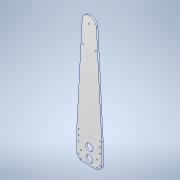
# Autodesk Inventor part: 関節3_側板1
Saved by Autodesk Inventor 2021 (Build 250183000, 183)
## iProperties
Created: 2022-01-31
Part Number: 関節3_側板1
Material: アルミニウム 6061
Document SubType Name: Modeling
Designer: hirohumi
Density: 2.7 g/cm^3
Appearance: アルミニウム - フラット
Author: hirohumi
Autodesk Inventor part; units mm, degrees
ref_plane "YZ Plane" through (0, 0, 0) normal (1, 0, 0) x (0, 1, 0)
ref_plane "XZ Plane" through (0, 0, 0) normal (0, 1, 0) x (-1, 0, 0)
ref_plane "XY Plane" through (0, 0, 0) normal (0, 0, 1) x (1, 0, 0)
sketch "スケッチ1" plane through (0, 0, 0) normal (0, 0, 1) x (1, 0, 0)
  circle A0 centre (0, 0) radius 10
  circle A1 centre (0, 0) radius 50 construction
  circle A2 centre (0, -28) radius 11.9375 construction
  circle A3 centre (-0.2119, 34.8748) radius 11.9375 construction
  circle A4 centre (0, -28) radius 15.9375 construction
  circle A5 centre (0, 0) radius 4 construction
  circle A6 centre (0, -28) radius 22.5 construction
  circle A7 centre (0, 300) radius 5 construction
  circle A8 centre (0, 300) radius 47.7465 construction
  line L0 (47.4611, 294.7873) -> (11.8661, -29.3033) construction
  line L1 (-47.4611, 294.7873) -> (-11.8661, -29.3033) construction
  circle A9 centre (-0.2119, 34.8748) radius 19.25 construction
  line L2 (-12.0776, 316.763) -> (11.6547, 316.763) construction
  line L3 (-22.6185, -92.0395) -> (22.1946, -92.0395) construction
  line L4 (22.5, -18) -> (-22.5, -18) construction
  line L5 (-22.5, -18) -> (-22.5, -38) construction
  line L6 (-22.5, -38) -> (22.5, -38) construction
  line L7 (22.5, -38) -> (22.5, -18) construction
  line L8 (22.5, -18) -> (-22.5, -38) construction
  line L9 (-22.5, -18) -> (22.5, -38) construction
  circle A10 centre (-22.5, -18) radius 1.6
  circle A11 centre (22.5, -18) radius 1.6
  circle A12 centre (22.5, -38) radius 1.6
  circle A13 centre (-22.5, -38) radius 1.6
  line L10 (30, 30) -> (-30, 30) construction
  line L11 (-30, 30) -> (-30, -30) construction
  line L12 (-30, -30) -> (30, -30) construction
  line L13 (30, -30) -> (30, 30) construction
  line L14 (30, 30) -> (-30, -30) construction
  line L15 (-30, 30) -> (30, -30) construction
  circle A14 centre (-30, 30) radius 1.25
  circle A15 centre (30, 30) radius 1.25
  circle A16 centre (30, -30) radius 1.25
  circle A17 centre (-30, -30) radius 1.25
  circle A18 centre (0, -28) radius 10
  circle A19 centre (0, 300) radius 1.75
  arc A20 (35, 30) -> (34.9923, 30.2769) centre (30, 30) ccw
  arc A21 (33.6477, -33.4197) -> (35, -30) centre (30, -30) ccw
  arc A22 (22.5, -43) -> (26.1477, -41.4197) centre (22.5, -38) ccw
  arc A23 (-26.1477, -41.4197) -> (-22.5, -43) centre (-22.5, -38) ccw
  arc A24 (-35, -30) -> (-33.6477, -33.4197) centre (-30, -30) ccw
  arc A25 (-34.9923, 30.2769) -> (-35, 30) centre (-30, 30) ccw
  arc A26 (19.9693, 301.1077) -> (-19.9693, 301.1077) centre (0, 300) ccw
  line L16 (-19.9693, 301.1077) -> (-34.9923, 30.2769)
  line L17 (-33.6477, -33.4197) -> (-26.1477, -41.4197)
  line L18 (19.9693, 301.1077) -> (34.9923, 30.2769)
  line L19 (33.6477, -33.4197) -> (26.1477, -41.4197)
  line L20 (22.5, -43) -> (-22.5, -43)
  circle A27 centre (-30, 0) radius 1.25
  circle A28 centre (30, 0) radius 1.25
  line L21 (-35, 30) -> (-35, -30)
  line L22 (35, -30) -> (35, 30)
  circle A29 centre (-30, 15) radius 1.6
  circle A30 centre (30, 15) radius 1.6
  circle A31 centre (-18, 242.7636) radius 1.6
  circle A32 centre (18, 242.7636) radius 1.6
  circle A33 centre (0, 300) radius 60 construction
  point P0 (0, 0)
  dimension "d0" = 20
  dimension "d1" = 100
  dimension "d11" = 23.875
  dimension "d12" = 23.875
  dimension "d16" = 8
  dimension "d17" = 45
  dimension "d18" = 28
  dimension "d19" = 4
  dimension "d26" = 10
  dimension "d27" = 300
  dimension "d28" = 95.493
  dimension "d30" = 38.5
  dimension "d36" = 45
  dimension "d37" = 20
  dimension "d38" = 3.2
  dimension "d39" = 3.2
  dimension "d40" = 3.2
  dimension "d41" = 3.2
  dimension "d46" = 60
  dimension "d47" = 60
  dimension "d48" = 2.5
  dimension "d49" = 2.5
  dimension "d50" = 2.5
  dimension "d51" = 2.5
  dimension "d52" = 20
  dimension "d53" = 3.5
  dimension "d55" = 5
  dimension "d56" = 5
  dimension "d57" = 20
  dimension "d58" = 5
  dimension "d59" = 5
  dimension "d60" = 5
  dimension "d61" = 5
  dimension "d64" = 2.5
  dimension "d65" = 2.5
  dimension "d66" = 3.2
  dimension "d67" = 3.2
  dimension "d68" = 15
  dimension "d69" = 3.2
  dimension "d70" = 3.2
  dimension "d71" = 120
  dimension "d72" = 36
  constraints: 46 end point, 34 centre point, 25 coincident, 21 point on circle, 15 tangent, 8 midpoint, 5 parallel, 4 horizontal, 4 horizontal alignment, 3 point on line, 2 perpendicular, 2 vertical alignment, 1 vertical
  measures "d0" diameter of A0
  measures "d1" diameter of A1
  measures "d11" diameter of A2
  measures "d12" diameter of A3
  measures "d16" diameter of A5
  measures "d17" diameter of A6
  measures "d18" distance of point (0, 0) A2.centre
  measures "d19" radial gap between concentric circles of A4 A2
  measures "d26" diameter of A7
  measures "d27" distance of point (0, 0) A7.centre
  measures "d28" diameter of A8
  measures "d30" diameter of A9
  measures "d36" distance of L6.end L5.end
  measures "d37" distance of L5.end L4.end
  measures "d38" diameter of A10
  measures "d39" diameter of A11
  measures "d40" diameter of A12
  measures "d41" diameter of A13
  measures "d46" distance of L12.end L11.end
  measures "d47" distance of L11.end L10.end
  measures "d48" diameter of A14
  measures "d49" diameter of A15
  measures "d50" diameter of A16
  measures "d51" diameter of A17
  measures "d52" diameter of A18
  measures "d53" diameter of A19
  measures "d55" radius of A20
  measures "d56" radius of A22
  measures "d57" radius of A26
  measures "d58" radius of A25
  measures "d59" radius of A24
  measures "d60" radius of A23
  measures "d61" radius of A21
  measures "d64" diameter of A27
  measures "d65" diameter of A28
  measures "d66" diameter of A29
  measures "d67" diameter of A30
  measures "d68" distance of A29.centre L10.end
  measures "d69" diameter of A31
  measures "d70" diameter of A32
  measures "d71" diameter of A33
  measures "d72" distance of A32.centre A31.centre
extrude "押し出し2" add sketch "スケッチ1" along normal blind 4
